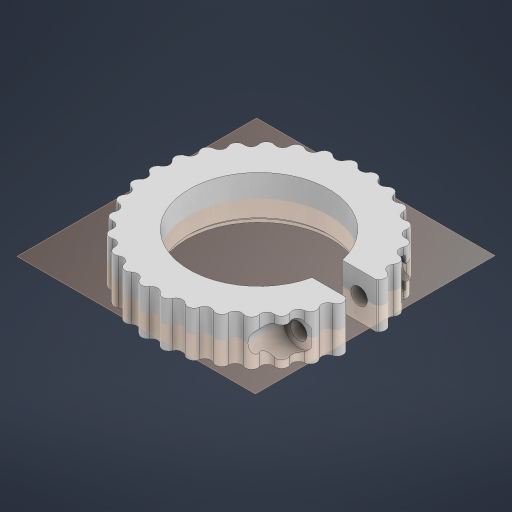
# Autodesk Inventor part: fastener
Saved by Autodesk Inventor 2024 (Build 280153000, 153)
## iProperties
Created: 2024-10-06
Part Number: fastener
Material: Generic
Document SubType Name: Modeling
Designer: loren
Density: 1 g/cm^3
Appearance: Default
Author: loren
## iProperties of the stored document fastener_3DPrint.ipt
Created: 2026-02-06
Part Number: fastener_3DPrint
Material: Generic
Document SubType Name: Modeling
Designer: lokies
Density: 1 g/cm^3
Appearance: Default
Author: lokies
Autodesk Inventor part; units mm, degrees
ref_plane "YZ Plane" through (0, 0, 0) normal (1, 0, 0) x (0, 1, 0)
ref_plane "XZ Plane" through (0, 0, 0) normal (0, 1, 0) x (-1, 0, 0)
ref_plane "XY Plane" through (0, 0, 0) normal (0, 0, 1) x (1, 0, 0)
sketch "Sketch1" plane through (0, 0, 0) normal (0, 1, 0) x (-1, 0, 0)
  line L0 (0, 0) -> (0, 6) construction
  line L1 (-9.65, 0) -> (-9.65, 0.4)
  line L2 (-9.65, 0.4) -> (-9.25, 0.8)
  line L3 (-9.25, 0.8) -> (-9.25, 6)
  line L4 (-9.25, 6) -> (-14.25, 6)
  line L5 (-14.25, 6) -> (-14.25, 0)
  line L6 (-14.25, 0) -> (-9.65, 0)
  dimension "d0" = 18.5
  dimension "d1" = 0.4
  dimension "d2" = 0.4
  dimension "d3" = 0.4
  dimension "d4" = 6
  dimension "d5" = 5
  constraints: 14 end point, 3 perpendicular, 2 point on line, 2 vertical, 1 parallel
  measures "d0" diameter of L3 L0
  measures "d1" distance from line of L1 L2.end
  measures "d2" horizontal distance of L1.end L2.end
  measures "d3" distance of L1.start L1.end
  measures "d4" distance between parallel lines of L6 L4
  measures "d5" distance between parallel lines of L5 L3
revolve "Revolution1" add sketch "Sketch1" angle 360 about axis through (0, 0, 0) along (0, 0, 1)
sketch "Sketch2" plane through (0, 0, 6) normal (0, 0, 1) x (1, 0, 0)
  circle A0 centre (0, 0) radius 14.25 projected
  arc A1 (-0.7011, 13.7955) -> (-1.4895, 14.1719) centre (-1.4022, 13.341) ccw
  arc A2 (1.4895, 14.1719) -> (0.7011, 13.7955) centre (1.4022, 13.341) ccw
  arc A3 (-0.7011, 13.7955) -> (0.7011, 13.7955) centre (0, 14.25) ccw
  point P0 (0, 0)
  dimension "d7" = 12
  constraints: 9 point on circle, 4 tangent, 3 centre point, 2 equal radius, 1 horizontal alignment
extrude "Extrusion1" cut sketch "Sketch2" against normal through all contours A2 A3 A1 A0 picked at (0, 13.9657)
pattern_circular "Circular Pattern1" count 30 over 360 about axis through (0, 0, -10) along (0, 0, 1) of "Extrusion1"
sketch "Sketch3" plane through (0, 13.25, 6) normal (0, 0, 1) x (1, 0, 0)
  circle A0 centre (0, -13.25) radius 9.25 projected
  line L0 (9.0312, -11.25) -> (19.0312, -11.25)
  line L1 (19.0312, -11.25) -> (19.0312, -15.25)
  line L2 (19.0312, -15.25) -> (9.0312, -15.25)
  line L3 (9.0312, -15.25) -> (9.0312, -11.25)
  circle A1 centre (0, -13.25) radius 9.25 projected
  dimension "d13" = 4
  dimension "d14" = 10
  constraints: 8 end point, 2 parallel, 2 point on circle, 1 horizontal, 1 perpendicular, 2 other
  measures "d13" distance between parallel lines of L2 L0
  measures "d14" distance between parallel lines of L1 L3
extrude "Extrusion2" cut sketch "Sketch3" against normal through all contours A0 L3 | A0 L0 L1 L2 picked at (9.0716, -13.6964)
ref_plane "Work Plane1" through (0, 14.25, 3) normal (0, 0, 1) x (1, 0, 0)
sketch "Sketch4" plane through (0, 14.25, 3) normal (0, 0, 1) x (1, 0, 0)
  line L0 (11.2708, 0.75) -> (11.2708, -29.25)
  line L1 (11.2708, 0.75) -> (12.3708, 0.75)
  line L2 (12.3708, 0.75) -> (12.3708, -20.25)
  line L3 (12.3708, -20.25) -> (13.2708, -20.25)
  line L4 (13.2708, -20.25) -> (13.2708, -29.25)
  line L5 (13.2708, -29.25) -> (11.2708, -29.25)
  line L6 (9.4405, -16.25) -> (13.5105, -16.25) projected
  line L7 (12.3708, -8.25) -> (12.4708, -8.25)
  line L8 (12.4708, -8.25) -> (12.4708, -6.55)
  line L9 (12.4708, -6.55) -> (12.3708, -6.55)
  line L10 (9.0312, -12.25) -> (13.5105, -12.25) projected
  point P0 (0, -14.25)
  point P1 (11.2708, -14.25)
  point P2 (12.3708, -9.75)
  point P3 (11.2708, -12.25)
  dimension "d17" = 30
  dimension "d18" = 2.2
  dimension "d19" = 4
  dimension "d20" = 4
  dimension "d21" = 1.7
  dimension "d22" = 0.1
  dimension "d23" = 4
  constraints: 18 end point, 4 perpendicular, 3 midpoint, 3 point on line, 2 horizontal, 2 vertical, 1 horizontal alignment, 1 parallel
  measures "d17" distance of L0.start L0.end
  measures "d18" diameter of point (12.371, -9.75) L0
  measures "d19" diameter of L4 L0
  measures "d20" distance between parallel lines of L6 L3
  measures "d21" distance of L7.end L8.end
  measures "d22" distance of L7.start L7.end
  measures "d23" distance between parallel lines of L7 L10
revolve "Revolution2" cut sketch "Sketch4" angle 360 about axis through (11.2708, 15, 3) along (0, -1, 0)
sketch "Sketch5" plane through (11.2708, 6, 3) normal (0, 1, 0) x (1, 0, 0)
  arc A0 (1.6182, 1.1753) -> (1.6182, -1.1753) centre (0, 0) ccw construction
  line L0 (2.3094, 0) -> (1.1547, -2)
  line L1 (1.1547, -2) -> (-1.1547, -2)
  line L2 (-1.1547, -2) -> (-2.3094, 0)
  line L3 (-2.3094, 0) -> (-1.1547, 2)
  line L4 (-1.1547, 2) -> (1.1547, 2)
  line L5 (1.1547, 2) -> (2.3094, 0)
  line L6 (1.1547, -2) -> (4, -2)
  line L7 (4, -2) -> (4, 2)
  line L8 (4, 2) -> (1.1547, 2)
  point P0 (-11.2708, 3)
  point P1 (1.6127, 1.1829)
  point P2 (1.6127, -1.1829)
  dimension "d25" = 4
  dimension "d28" = 4
  constraints: 18 end point, 2 horizontal, 1 coincident, 1 collinear, 1 perpendicular, 13 other
  measures "d25" distance between parallel lines of L4 L1
  measures "d28" distance from line of point (0, 0) L7
extrude "Extrusion3" cut sketch "Sketch5" along normal up to surface (1.7 mm away)
equation "\"d2\" = d1"
equation "\"d3\" = d2"
equation "\"d23\" = d20"
equation "\"d28\" = d25"
body "Solid1"
